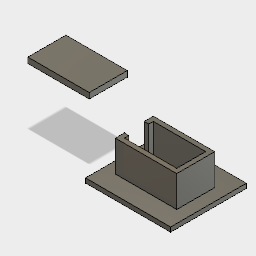
Servo Stand (Autodesk Fusion 360 design; units mm, degrees)
Autodesk Fusion 360 part; units mm, degrees
sketch "Sketch1" plane through (0, 0, 0) normal (0, 1, 0) x (1, 0, 0)
  line L0 (0, 30) -> (22.74, 30)
  line L1 (22.74, 30) -> (22.74, 17.43)
  line L2 (22.74, 17.43) -> (0, 17.43)
  line L3 (0, 17.43) -> (0, 30)
  line L4 (22.24, 17.93) -> (0.5, 17.93)
  line L5 (0.5, 17.93) -> (0.5, 29.5)
  line L6 (0.5, 29.5) -> (22.24, 29.5)
  line L7 (22.24, 29.5) -> (22.24, 17.93)
  dimension "d1" = 22.74
  dimension "d2" = 12.57
  dimension "d3" = 0.5
  measures "d1" distance of L0.start L0.end
  measures "d2" distance of L0.start L2.end
extrude "Extrude1" add sketch "Sketch1" along normal blind 14 contours L0 L1 L2 L3 | L4 L5 L6 L7 makes body 1
shell "Shell1" thickness 2 outward yes removed faces 0 bodies 1
ref_plane "WorkPlane1" through (11.37, 13.5, -23.715) normal (0, 1, 0) x (0, 0, 1)
split "Split1" by plane through (11.37, 13.5, -23.715) normal (0, 1, 0) bodies 1 makes body 2 at (6.9133, 16, -20.9533)
move_body "Move1" bodies 2 to x (1, 0, 0) y (0, 1, 0) z (0, 0, 1) at (-38, 9, 0)
sketch "Sketch2" plane through (-2, 0, 0) normal (-1, 0, 0) x (0, 0, 1)
  line L0 (-15.43, 13.5) -> (-32, 13.5)
  line L1 (-32, 13.5) -> (-32, -2)
  line L2 (-32, -2) -> (-15.43, -2)
  line L3 (-15.43, -2) -> (-15.43, 13.5)
  line L4 (-28.0144, 13.5) -> (-19.4144, 13.5)
  line L5 (-19.4144, 13.5) -> (-19.4144, 2)
  line L6 (-19.4144, 2) -> (-28.0144, 2)
  line L7 (-28.0144, 2) -> (-28.0144, 13.5)
  dimension "d8" = 8.6
  measures "d8" distance of L4.start L4.end
extrude "Extrude2" cut sketch "Sketch2" against normal blind 5 contours L0 L4 L5 L6 L7 bodies 1
sketch "Sketch3" plane through (0, 0, -17.43) normal (0, 0, -1) x (-1, 0, 0)
  line L0 (0, 13.5) -> (-22.74, 13.5)
  line L1 (-22.74, 13.5) -> (-22.74, 0)
  line L2 (-22.74, 0) -> (0, 0)
  line L3 (0, 0) -> (0, 13.5)
sketch "Sketch4" plane through (0, 0, 0) normal (0, 1, 0) x (1, 0, 0)
  line L0 (-2, 9.9798) -> (35, 9.9798)
  line L1 (35, 9.9798) -> (35, -23)
  line L2 (35, -23) -> (-2, -23)
  line L3 (-2, -23) -> (-2, 9.9798)
  dimension "d11" = 37
  measures "d11" distance of L0.start L0.end
extrude "Extrude3" add sketch "Sketch4" along normal blind 2 separate body makes body 3
move_body "Move2" bodies 3 to x (1, 0, 0) y (0, 1, 0) z (0, 0, 1) at (-5, -2, -30.5)
combine "Combine1" operation add target body 1 tool bodies 3
